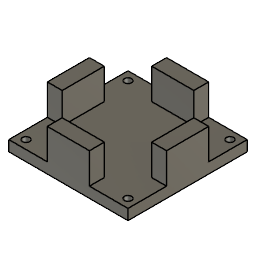
cubeHolderCap (Autodesk Fusion 360 design; units mm, degrees)
part number: 2026-03-05-11-06-03-534
Autodesk Fusion 360 part; units mm, degrees
sketch "Sketch1" plane through (0, 0, 0) normal (0, 0, 1) x (1, 0, 0)
  line L0 (28, 28) -> (-28, 28)
  line L1 (-28, 28) -> (-28, -28)
  line L2 (-28, -28) -> (28, -28)
  line L3 (28, -28) -> (28, 28)
  line L4 (28, 28) -> (-28, -28) construction
  line L5 (-28, 28) -> (28, -28) construction
  line L6 (21, 21) -> (-21, 21)
  line L7 (-21, 21) -> (-21, -21)
  line L8 (-21, -21) -> (21, -21)
  line L9 (21, -21) -> (21, 21)
  line L10 (21, 21) -> (-21, -21) construction
  line L11 (-21, 21) -> (21, -21) construction
  line L12 (-28, 0) -> (28, 0) construction
  line L13 (0, 28) -> (0, -28) construction
  line L14 (-28, 9.9) -> (-21, 9.9)
  line L15 (-21, 9.9) -> (-21, -9.9)
  line L16 (-21, -9.9) -> (-28, -9.9)
  line L17 (-28, -9.9) -> (-28, 9.9)
  line L18 (21, -9.9) -> (28, -9.9)
  line L19 (28, 9.9) -> (21, 9.9)
  line L20 (-9.9, -28) -> (9.9, -28)
  line L21 (9.9, -28) -> (9.9, -21)
  line L22 (9.9, -21) -> (-9.9, -21)
  line L23 (-9.9, -21) -> (-9.9, -28)
  line L24 (9.9, 28) -> (9.9, 21)
  line L25 (-9.9, 21) -> (-9.9, 28)
  circle A0 centre (23.94, 23.94) radius 1.7
  circle A1 centre (-23.94, 23.94) radius 1.7
  circle A2 centre (23.94, -23.94) radius 1.7
  circle A3 centre (-23.94, -23.94) radius 1.7
  dimension "d1" = 56
  dimension "d2" = 56
  dimension "d3" = 42
  dimension "d4" = 42
  dimension "d5" = 19.8
  dimension "d6" = 19.8
  dimension "d7" = 3.4
  dimension "d8" = 4.06
  dimension "d9" = 7
  constraint horizontal L0
  constraint perpendicular L0 L1
  constraint parallel L0 L2
  constraint parallel L1 L3
  constraint coincident L4 origin
  constraint coincident L5 origin
  constraint horizontal L6
  constraint perpendicular L6 L7
  constraint parallel L6 L8
  constraint parallel L7 L9
  constraint coincident L10 origin
  constraint coincident L11 origin
  constraint coincident L1 L12.start
  constraint coincident L3 L12.end
  constraint perpendicular L3 L12
  constraint midpoint origin L12
  constraint midpoint L0 L13.start
  constraint midpoint L2 L13.end
  constraint horizontal L14
  constraint vertical L15
  constraint horizontal L16
  constraint vertical L17
  constraint coincident L1 L14.start
  constraint midpoint L12.start L17
  constraint coincident L7 L15.end
  constraint symmetric L13 L14.start L19.start
  constraint symmetric L13 L14.end L19.end
  constraint symmetric L13 L15.end L18.start
  constraint symmetric L13 L16.end L18.end
  constraint horizontal L20
  constraint vertical L21
  constraint horizontal L22
  constraint vertical L23
  constraint coincident L8 L21.end
  constraint coincident L2 L20.start
  constraint midpoint L13.end L20
  constraint symmetric L12 L20.start L25.end
  constraint symmetric L12 L20.end L24.start
  constraint symmetric L12 L21.end L24.end
  constraint symmetric L12 L22.end L25.start
  constraint coincident L4 A0.centre
  constraint symmetric L13 A0 A1
  constraint symmetric L12 A0 A2
  constraint symmetric L12 A1 A3
  measures "d1" distance of L1.end L2.end
  measures "d2" distance of L0.end L1.end
  measures "d3" distance of L7.end L8.end
  measures "d4" distance of L6.end L7.end
  measures "d5" distance of L14.start L16.end
  measures "d6" distance of L21 L23
  measures "d7" diameter of A0
  measures "d8" vertical distance of L0.start A0.centre
  measures "d9" distance of L1 L7
sketch "Sketch2" plane through (0, 0, 0) normal (0, 1, 0) x (1, 0, 0)
  point P0 (0, -5)
  point P1 (0, -19.4)
  dimension "d10" = 5
  dimension "d11" = 14.4
  constraint vertical P0 P1
  constraint vertical P1 origin
  measures "d10" distance of P0 origin
  measures "d11" distance of P0 P1
extrude "Extrude1" add sketch "Sketch1" along normal up to surface (5 mm away)
extrude "Extrude2" add sketch "Sketch1" along normal up to surface (14.4 mm away) from surface at 5 contours L0 L6 L24 L25 | L3 L9 L18 L19 | L1 L7 L14 L15 L16 L17 | L2 L8 L20 L21 L22 L23
equation "d6 = d5"
equation "d8 = 0.29 * ( d1 - d3 )"
